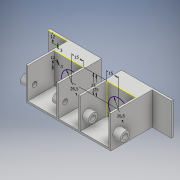
# Autodesk Inventor part: Chassi_Rear
Saved by Autodesk Inventor 2018.2 (Build 222227000, 227)
## iProperties
Created: 2018-08-12
Part Number: Chassi_Rear
Material: Generic
Document SubType Name: Modeling
Designer: mateu
Density: 1 g/cm^3
Appearance: Default
Author: mateu
Autodesk Inventor part; units mm, degrees
ref_plane "YZ Plane" through (0, 0, 0) normal (1, 0, 0) x (0, 1, 0)
ref_plane "XZ Plane" through (0, 0, 0) normal (0, 1, 0) x (-1, 0, 0)
ref_plane "XY Plane" through (0, 0, 0) normal (0, 0, 1) x (1, 0, 0)
sketch "Sketch1" plane through (0, 0, 0) normal (0, 0, 1) x (1, 0, 0)
  line L0 (0, 0) -> (110, 0)
  line L1 (110, 0) -> (110, -56)
  line L2 (110, -56) -> (0, -56)
  line L3 (0, -56) -> (0, 0)
  line L4 (0, 0) -> (-25, 0)
  line L5 (-25, 0) -> (-25, -2.4)
  line L6 (-25, -2.4) -> (0, -2.4)
  line L7 (0, -2.4) -> (0, 0)
  line L8 (110, 0) -> (135, 0)
  line L9 (135, 0) -> (135, -2.4)
  line L10 (135, -2.4) -> (110, -2.4)
  line L11 (110, -2.4) -> (110, 0)
  dimension "d0" = 110
  dimension "d1" = 56
  dimension "d2" = 25
  dimension "d3" = 2.4
  dimension "d4" = 25
  dimension "d5" = 2.4
  constraints: 24 end point, 6 parallel, 3 horizontal, 3 perpendicular
  measures "d0" distance of L1.end L2.end
  measures "d1" distance of L0.end L1.end
  measures "d2" distance of L6.end L5.end
  measures "d3" distance of L5.end L4.end
  measures "d4" distance of L9.end L10.end
  measures "d5" distance of L8.end L9.end
extrude "Extrusion1" add sketch "Sketch1" along normal blind 42
sketch "Sketch2" plane through (0, 0, 42) normal (0, 0, 1) x (1, 0, 0)
  line L0 (2.4, -2.4) -> (107.6, -2.4)
  line L1 (107.6, -2.4) -> (107.6, -54.7735)
  line L2 (2.4, -54.7735) -> (2.4, -2.4)
  line L3 (110, -56) -> (110, -2.4) projected
  line L4 (0, -2.4) -> (0, -56) projected
  line L5 (107.6, -54.7735) -> (107.6, -56)
  line L6 (2.4, -54.7735) -> (2.4, -56)
  line L7 (0, -56) -> (110, -56) projected
  point P0 (0, 0)
  dimension "d8" = 2.4
  dimension "d9" = 2.4
  constraints: 10 end point, 2 vertical, 1 horizontal, 1 parallel, 1 perpendicular, 1 point on line
  measures "d8" distance between parallel lines of L3 L1
  measures "d9" distance between parallel lines of L4 L2
extrude "Extrusion2" cut sketch "Sketch2" against normal blind 39.6
sketch "Sketch3" plane through (0, 0, 42) normal (0, 0, 1) x (1, 0, 0)
  line L0 (135, 0) -> (-25, 0) projected
  line L1 (55, 0) -> (68, 0)
  line L2 (55, 0) -> (42, 0)
  line L3 (42, 0) -> (42, -2.4)
  line L4 (2.4, -2.4) -> (107.6, -2.4) projected
  line L5 (68, -2.4) -> (42, -2.4)
  line L6 (68, -2.4) -> (68, 0)
  point P0 (0, 0)
  dimension "d12" = 13
  dimension "d13" = 13
  constraints: 10 end point, 4 point on line, 2 perpendicular, 1 collinear, 1 midpoint
  measures "d12" distance of L1.start L1.end
  measures "d13" distance of L1.start L2.end
extrude "Extrusion3" cut sketch "Sketch3" against normal blind 39.6
sketch "Sketch4" plane through (0, 0, 2.4) normal (0, 0, 1) x (1, 0, 0)
  line L0 (2.4, -2.4) -> (42, -2.4) projected
  line L1 (107.6, -56) -> (2.4, -56) projected
  line L2 (42, -2.4) -> (39.6, -2.4)
  line L3 (39.6, -2.4) -> (39.6, -56)
  line L4 (39.6, -56) -> (42, -56)
  line L5 (42, -56) -> (42, -2.4)
  line L6 (68, -2.4) -> (107.6, -2.4) projected
  line L7 (68, -2.4) -> (70.4, -2.4)
  line L8 (70.4, -2.4) -> (70.4, -56)
  line L9 (70.4, -56) -> (68, -56)
  line L10 (68, -56) -> (68, -2.4)
  point P0 (0, 0)
  dimension "d16" = 2.4
  dimension "d17" = 2.4
  constraints: 16 end point, 4 parallel, 2 horizontal, 2 perpendicular, 2 point on line
  measures "d16" distance of L4.end L3.end
  measures "d17" distance of L8.end L9.end
extrude "Extrusion4" add sketch "Sketch4" along normal blind 39.6
sketch "Sketch5" plane through (-25, -2.4, 0) normal (0, -1, 0) x (1, 0, 0)
  circle A0 centre (12.5, 30) radius 1.5
  circle A1 centre (12.5, 12) radius 1.5
  line L0 (0, 42) -> (25, 42) projected
  line L1 (0, 0) -> (25, 0) projected
  dimension "d20" = 3
  dimension "d21" = 3
  dimension "d22" = 12
  dimension "d23" = 12
  constraints: 2 centre point
  measures "d20" diameter of A0
  measures "d21" diameter of A1
  measures "d22" distance from line of L0 A0.centre
  measures "d23" distance from line of L1 A1.centre
sketch "Sketch6" plane through (2.4, -2.4, 2.4) normal (0, -1, 0) x (1, 0, 0)
  line L0 (37.2, 0) -> (37.2, 39.6) projected
  line L1 (0, 39.6) -> (37.2, 39.6)
  line L2 (37.2, 39.6) -> (37.2, 0)
  line L3 (37.2, 0) -> (0, 0)
  line L4 (0, 0) -> (0, 39.6)
  line L5 (68, 39.6) -> (68, 0) projected
  line L6 (105.2, 39.6) -> (105.2, 0) projected
  line L7 (68, 39.6) -> (105.2, 39.6)
  line L8 (105.2, 39.6) -> (105.2, 0)
  line L9 (105.2, 0) -> (68, 0)
  line L10 (68, 0) -> (68, 39.6)
  point P0 (-2.4, -2.4)
  constraints: 16 end point, 4 parallel, 2 horizontal, 2 perpendicular
extrude "Extrusion5" add sketch "Sketch6" along normal blind 19
sketch "Sketch7" plane through (0, -56, 0) normal (-1, 0, 0) x (0, 0, 1)
  circle A0 centre (17, 8.6) radius 3.15
  line L0 (0, 53.6) -> (0, 0) projected
  line L1 (0, 53.6) -> (42, 53.6) projected
  point P0 (0, 56)
  dimension "d26" = 6.3
  dimension "d27" = 17
  dimension "d28" = 45
  constraints: 1 centre point
  measures "d26" diameter of A0
  measures "d27" distance from line of L0 A0.centre
  measures "d28" distance from line of L1 A0.centre
extrude "Extrusion6" cut sketch "Sketch7" against normal blind 110
sketch "Sketch8" plane through (0, -56, 0) normal (-1, 0, 0) x (0, 0, 1)
  circle A0 centre (17, 8.6) radius 3.15 projected
  circle A1 centre (17, 8.6) radius 6
  point P0 (0, 56)
  dimension "d31" = 12
  constraints: 1 centre point, 1 coincident
  measures "d31" diameter of A1
extrude "Extrusion7" add sketch "Sketch8" along normal blind 10
sketch "Sketch9" plane through (39.6, -56, 2.4) normal (-1, 0, 0) x (0, 0, 1)
  circle A0 centre (14.6, 8.6) radius 3.15 projected
  circle A1 centre (14.6, 8.6) radius 6
  point P0 (-2.4, 56)
  dimension "d34" = 12
  constraints: 1 centre point, 1 coincident
  measures "d34" diameter of A1
extrude "Extrusion8" add sketch "Sketch9" along normal blind 8
sketch "Sketch10" plane through (110, -56, 0) normal (1, 0, 0) x (0, 0, -1)
  circle A0 centre (-17, 8.6) radius 3.15 projected
  circle A1 centre (-17, 8.6) radius 6
  point P0 (0, 56)
  dimension "d37" = 12
  constraints: 1 centre point, 1 coincident
  measures "d37" diameter of A1
extrude "Extrusion9" add sketch "Sketch10" along normal blind 10
sketch "Sketch11" plane through (70.4, -56, 42) normal (1, 0, 0) x (0, 0, -1)
  circle A0 centre (25, 8.6) radius 3.15 projected
  circle A1 centre (25, 8.6) radius 6
  point P0 (42, 56)
  dimension "d40" = 12
  constraints: 1 centre point, 1 coincident
  measures "d40" diameter of A1
extrude "Extrusion10" add sketch "Sketch11" along normal blind 8
sketch "Sketch12" plane through (2.4, -21.4, 2.4) normal (0, -1, 0) x (1, 0, 0)
  circle A0 centre (22.2, 14.6) radius 13.25
  circle A1 centre (83, 14.6) radius 13.25
  line L0 (68, 0) -> (68, 39.6) projected
  line L1 (37.2, 0) -> (37.2, 39.6) projected
  line L2 (37.2, 39.6) -> (0, 39.6) projected
  line L3 (105.2, 39.6) -> (68, 39.6) projected
  point P0 (-2.4, -2.4)
  dimension "d43" = 26.5
  dimension "d44" = 26.5
  dimension "d45" = 15
  dimension "d46" = 15
  dimension "d47" = 25
  dimension "d48" = 25
  constraints: 2 centre point
  measures "d43" diameter of A0
  measures "d44" diameter of A1
  measures "d45" distance from line of L0 A1.centre
  measures "d46" distance from line of L1 A0.centre
  measures "d47" distance from line of L2 A0.centre
  measures "d48" distance from line of L3 A1.centre
body "Solid1"
